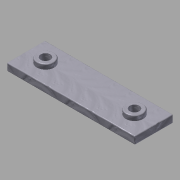
# Autodesk Inventor part: CIM MountBase
Saved by Autodesk Inventor 2013 (Build 170138000, 138)
## iProperties
Created: 2013-01-18
Part Number: CIM MountBase
Material: Aluminum 6061, Welded
Document SubType Name: Modeling
Designer: Naphat
Density: 1 g/cm^3
Author: Naphat
Autodesk Inventor part; units mm, degrees
ref_plane "YZ Plane" through (0, 0, 0) normal (1, 0, 0) x (0, 1, 0)
ref_plane "XZ Plane" through (0, 0, 0) normal (0, 1, 0) x (-1, 0, 0)
ref_plane "XY Plane" through (0, 0, 0) normal (0, 0, 1) x (1, 0, 0)
sketch "Sketch1" plane through (0, 0, 0) normal (0, 1, 0) x (-1, 0, 0)
  line L0 (0, 0) -> (112, 0)
  line L1 (112, 0) -> (112, 40)
  line L2 (112, 40) -> (0, 40)
  line L3 (0, 40) -> (0, 0)
  circle A0 centre (9.4996, 20) radius 5
  circle A1 centre (102.489, 20) radius 5
  dimension "d0" = 112
  dimension "d1" = 40
  dimension "d4" = 10
  dimension "d5" = 10
  dimension "d18" = 92.9894
  dimension "d19" = 9.4996
  dimension "d22" = 9.511
  dimension "d23" = 40
  dimension "d24" = 20
  constraints: 8 end point, 2 centre point, 2 perpendicular, 1 horizontal, 1 parallel
  measures "d0" distance of L0.start L0.end
  measures "d1" distance of L0.end L1.end
  measures "d4" diameter of A0
  measures "d5" diameter of A1
  measures "d18" distance of A1.centre A0.centre
  measures "d19" distance from line of A0.centre L3
  measures "d22" distance from line of A1.centre L1
  measures "d23" distance of L2.end L0.start
  measures "d24" distance from line of L2 A0.centre
extrude "Extrusion1" add sketch "Sketch1" along normal blind 8
sketch "Sketch2" plane through (0, 8, 0) normal (0, 1, 0) x (1, 0, 0)
  circle A0 centre (-102.489, -20) radius 5 projected
  circle A1 centre (-9.4996, -20) radius 5 projected
  circle A2 centre (-102.489, -20) radius 9
  circle A3 centre (-9.4996, -20) radius 9
  dimension "d8" = 18
  dimension "d9" = 18
  constraints: 2 centre point, 2 coincident
  measures "d8" diameter of A2
  measures "d9" diameter of A3
extrude "Extrusion2" add sketch "Sketch2" along normal blind 5
sketch "Sketch3" plane through (-112, 0, 0) normal (-1, 0, 0) x (0, 0, 1)
  line L0 (0, 0) -> (40, 0) projected
  line L1 (40, 0) -> (40, 8) projected
  line L2 (0, 8) -> (40, 8) projected
  line L3 (0, 0) -> (0, 8) projected
extrude "Extrusion3" add sketch "Sketch3" along normal blind 11
sketch "Sketch4" plane through (0, 0, 40) normal (1, 0, 0) x (0, 0, -1)
  line L0 (0, 0) -> (40, 0) projected
  line L1 (40, 0) -> (40, 8) projected
  line L2 (0, 8) -> (40, 8) projected
  line L3 (0, 0) -> (0, 8) projected
extrude "Extrusion4" add sketch "Sketch4" along normal blind 11
fillet "Fillet1" radius 1 13 edges at (-123, 4, 40) (-56, 0, 40) (-56, 0, 0) (-123, 0, 20) (11, 0, 20) (11, 4, 40) (11, 4, 0) (-56, 8, 0) (11, 8, 20) (-56, 8, 40) (-123, 8, 20) (-111.489, 13, 20) (-18.4996, 13, 20)
equation "\"d5\" = d4"
equation "\"d24\" = 0.5 * d23"
equation "\"d9\" = d8"
body "Solid1"
